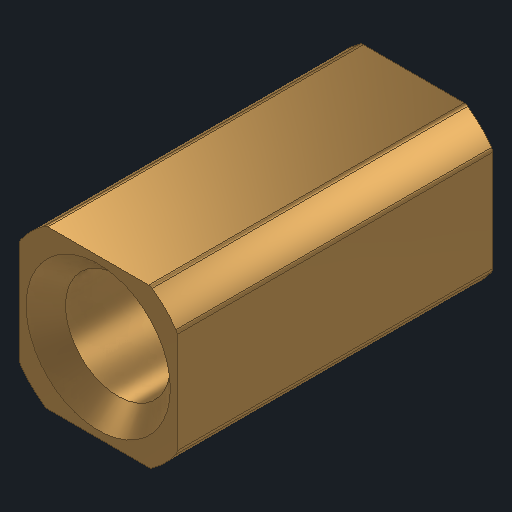
# Autodesk Inventor part: HS Shaft Adapter Circle
Saved by Autodesk Inventor 2026.2 (Build 302298000, 298)
## iProperties
Created: 2022-08-02
Part Number: HS Shaft Adapter Circle
Material: Generic
Document SubType Name: Modeling
Designer: ylu12
Density: 1 g/cm^3
Appearance: Sintered Bronze
Author: ylu12
Autodesk Inventor part; units mm, degrees
ref_plane "YZ Plane" through (0, 0, 0) normal (1, 0, 0) x (0, 1, 0)
ref_plane "XZ Plane" through (0, 0, 0) normal (0, 1, 0) x (-1, 0, 0)
ref_plane "XY Plane" through (0, 0, 0) normal (0, 0, 1) x (1, 0, 0)
sketch "Sketch1" plane through (0, 0, 0) normal (0, 0, 1) x (1, 0, 0)
  line L0 (-3.175, -3.175) -> (3.175, -3.175)
  line L1 (3.175, -3.175) -> (3.175, 3.175)
  line L2 (3.175, 3.175) -> (-3.175, 3.175)
  line L3 (-3.175, 3.175) -> (-3.175, -3.175)
  line L4 (-3.175, -3.175) -> (3.175, 3.175) construction
  line L5 (3.175, -3.175) -> (-3.175, 3.175) construction
  circle A0 centre (0, 0) radius 3.81
  point P0 (2.1061, -3.175)
  point P1 (3.175, -2.1061)
  point P2 (3.175, 2.1061)
  point P3 (2.1061, 3.175)
  point P4 (-2.1061, 3.175)
  point P5 (-3.175, 2.1061)
  point P6 (-3.175, -2.1061)
  point P7 (-2.1061, -3.175)
  dimension "d0" = 7.62
  dimension "d1" = 6.35
  constraints: 12 end point, 2 midpoint, 2 parallel, 2 perpendicular, 1 centre point, 1 coincident, 1 horizontal
  measures "d0" diameter of A0
  measures "d1" distance between parallel lines of L2 L0
extrude "Extrusion1" add sketch "Sketch1" against normal blind 12.7 contours A0 L3 L2 L1 L0
sketch "Sketch2" plane through (0, 0, 0) normal (0, 0, 1) x (1, 0, 0)
  arc A0 (2.1061, -3.175) -> (3.175, -2.1061) centre (0, 0) ccw construction
  circle A1 centre (0, 0) radius 2.1082
  dimension "d4" = 4.2164
  constraints: 1 centre point, 1 coincident
  measures "d4" diameter of A1
extrude "Extrusion2" cut sketch "Sketch2" against normal blind 12.7
fillet "Fillet1" radius 0.254 8 edges at (2.1061, 3.175, -6.35) (3.175, 2.1061, -6.35) (3.175, -2.1061, -6.35) (2.1061, -3.175, -6.35) (-2.1061, -3.175, -6.35) (-3.175, -2.1061, -6.35) (-3.175, 2.1061, -6.35) (-2.1061, 3.175, -6.35)
chamfer "Chamfer1" distance 0.7937 angle 45 2 edges at (-2.1082, 0, 0) (-2.1082, 0, -12.7)
body "Solid1"
